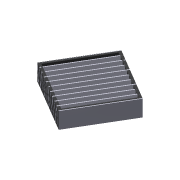
# Autodesk Inventor part: filter ver1
Saved by Autodesk Inventor 2016 (Build 200138000, 138)
## iProperties
Created: 2018-02-22
Part Number: filter ver1
Material: Generic
Document SubType Name: Modeling
Designer: Juny
Density: 1 g/cm^3
Appearance: Default
Author: Juny
Autodesk Inventor part; units mm, degrees
ref_plane "YZ Plane" through (0, 0, 0) normal (1, 0, 0) x (0, 1, 0)
ref_plane "XZ Plane" through (0, 0, 0) normal (0, 1, 0) x (-1, 0, 0)
ref_plane "XY Plane" through (0, 0, 0) normal (0, 0, 1) x (1, 0, 0)
sketch "Sketch1" plane through (0, 0, 0) normal (0, 0, 1) x (1, 0, 0)
  line L0 (22.5214, 7.9449) -> (30.3551, 21.1573) projected
  ellipse E0 centre (32.9355, 19.6263) end of major axis (32.1925, 22.5337) minor radius 3 (34.465, 22.2076) -> (30.3551, 21.1573) ccw projected
  line L1 (34.465, 22.2076) -> (47.6774, 14.3739) projected
  ellipse E1 centre (46.1463, 11.7935) end of major axis (49.0538, 12.5365) minor radius 3 (48.7277, 10.264) -> (47.6774, 14.3739) ccw projected
  line L2 (48.7277, 10.264) -> (40.894, -2.9483) projected
  ellipse E2 centre (38.3136, -1.4173) end of major axis (39.0566, -4.3248) minor radius 3 (36.7841, -3.9987) -> (40.894, -2.9483) ccw projected
  line L3 (36.7841, -3.9987) -> (23.5717, 3.835) projected
  ellipse E3 centre (25.1028, 6.4154) end of major axis (22.1953, 5.6724) minor radius 3 (22.5214, 7.9449) -> (23.5717, 3.835) ccw projected
  line L4 (9.2613, -14.4196) -> (17.095, -1.2072) projected
  ellipse E4 centre (19.6755, -2.7383) end of major axis (18.9324, 0.1692) minor radius 3 (21.2049, -0.1569) -> (17.095, -1.2072) ccw projected
  line L5 (21.2049, -0.1569) -> (34.4173, -7.9906) projected
  ellipse E5 centre (32.8863, -10.571) end of major axis (35.7938, -9.828) minor radius 3 (35.4677, -12.1005) -> (34.4173, -7.9906) ccw projected
  line L6 (35.4677, -12.1005) -> (27.634, -25.3129) projected
  ellipse E6 centre (25.0535, -23.7818) end of major axis (25.7966, -26.6893) minor radius 3 (23.5241, -26.3632) -> (27.634, -25.3129) ccw projected
  line L7 (23.5241, -26.3632) -> (10.3117, -18.5295) projected
  ellipse E7 centre (11.8427, -15.9491) end of major axis (8.9353, -16.6921) minor radius 3 (9.2613, -14.4196) -> (10.3117, -18.5295) ccw projected
  line L8 (-3.9987, -36.7841) -> (3.835, -23.5717) projected
  ellipse E8 centre (6.4154, -25.1028) end of major axis (5.6724, -22.1953) minor radius 3 (7.9449, -22.5214) -> (3.835, -23.5717) ccw projected
  line L9 (7.9449, -22.5214) -> (21.1573, -30.3551) projected
  ellipse E9 centre (19.6263, -32.9355) end of major axis (22.5337, -32.1925) minor radius 3 (22.2076, -34.465) -> (21.1573, -30.3551) ccw projected
  line L10 (22.2076, -34.465) -> (14.3739, -47.6774) projected
  ellipse E10 centre (11.7935, -46.1463) end of major axis (12.5365, -49.0538) minor radius 3 (10.264, -48.7277) -> (14.3739, -47.6774) ccw projected
  line L11 (10.264, -48.7277) -> (-2.9483, -40.894) projected
  ellipse E11 centre (-1.4173, -38.3136) end of major axis (-4.3248, -39.0566) minor radius 3 (-3.9987, -36.7841) -> (-2.9483, -40.894) ccw projected
  line L12 (0.1569, 21.2049) -> (7.9906, 34.4173) projected
  ellipse E12 centre (10.571, 32.8863) end of major axis (9.828, 35.7938) minor radius 3 (12.1005, 35.4677) -> (7.9906, 34.4173) ccw projected
  line L13 (12.1005, 35.4677) -> (25.3129, 27.634) projected
  ellipse E13 centre (23.7818, 25.0535) end of major axis (26.6893, 25.7966) minor radius 3 (26.3632, 23.5241) -> (25.3129, 27.634) ccw projected
  line L14 (26.3632, 23.5241) -> (18.5295, 10.3117) projected
  ellipse E14 centre (15.9491, 11.8427) end of major axis (16.6921, 8.9353) minor radius 3 (14.4196, 9.2613) -> (18.5295, 10.3117) ccw projected
  line L15 (14.4196, 9.2613) -> (1.2072, 17.095) projected
  ellipse E15 centre (2.7383, 19.6755) end of major axis (-0.1692, 18.9324) minor radius 3 (0.1569, 21.2049) -> (1.2072, 17.095) ccw projected
  line L16 (-13.1032, -1.1596) -> (-5.2695, 12.0528) projected
  ellipse E16 centre (-2.689, 10.5218) end of major axis (-3.4321, 13.4293) minor radius 3 (-1.1596, 13.1032) -> (-5.2695, 12.0528) ccw projected
  line L17 (-1.1596, 13.1032) -> (12.0528, 5.2695) projected
  ellipse E17 centre (10.5218, 2.689) end of major axis (13.4293, 3.4321) minor radius 3 (13.1032, 1.1596) -> (12.0528, 5.2695) ccw projected
  line L18 (13.1032, 1.1596) -> (5.2695, -12.0528) projected
  ellipse E18 centre (2.689, -10.5218) end of major axis (3.4321, -13.4293) minor radius 3 (1.1596, -13.1032) -> (5.2695, -12.0528) ccw projected
  line L19 (1.1596, -13.1032) -> (-12.0528, -5.2695) projected
  ellipse E19 centre (-10.5218, -2.689) end of major axis (-13.4293, -3.4321) minor radius 3 (-13.1032, -1.1596) -> (-12.0528, -5.2695) ccw projected
  line L20 (-26.3632, -23.5241) -> (-18.5295, -10.3117) projected
  ellipse E20 centre (-15.9491, -11.8427) end of major axis (-16.6921, -8.9353) minor radius 3 (-14.4196, -9.2613) -> (-18.5295, -10.3117) ccw projected
  line L21 (-14.4196, -9.2613) -> (-1.2072, -17.095) projected
  ellipse E21 centre (-2.7383, -19.6755) end of major axis (0.1692, -18.9324) minor radius 3 (-0.1569, -21.2049) -> (-1.2072, -17.095) ccw projected
  line L22 (-0.1569, -21.2049) -> (-7.9906, -34.4173) projected
  ellipse E22 centre (-10.571, -32.8863) end of major axis (-9.828, -35.7938) minor radius 3 (-12.1005, -35.4677) -> (-7.9906, -34.4173) ccw projected
  line L23 (-12.1005, -35.4677) -> (-25.3129, -27.634) projected
  ellipse E23 centre (-23.7818, -25.0535) end of major axis (-26.6893, -25.7966) minor radius 3 (-26.3632, -23.5241) -> (-25.3129, -27.634) ccw projected
  line L24 (-22.2076, 34.465) -> (-14.3739, 47.6774) projected
  ellipse E24 centre (-11.7935, 46.1463) end of major axis (-12.5365, 49.0538) minor radius 3 (-10.264, 48.7277) -> (-14.3739, 47.6774) ccw projected
  line L25 (-10.264, 48.7277) -> (2.9483, 40.894) projected
  ellipse E25 centre (1.4173, 38.3136) end of major axis (4.3248, 39.0566) minor radius 3 (3.9987, 36.7841) -> (2.9483, 40.894) ccw projected
  line L26 (3.9987, 36.7841) -> (-3.835, 23.5717) projected
  ellipse E26 centre (-6.4154, 25.1028) end of major axis (-5.6724, 22.1953) minor radius 3 (-7.9449, 22.5214) -> (-3.835, 23.5717) ccw projected
  line L27 (-7.9449, 22.5214) -> (-21.1573, 30.3551) projected
  ellipse E27 centre (-19.6263, 32.9355) end of major axis (-22.5337, 32.1925) minor radius 3 (-22.2076, 34.465) -> (-21.1573, 30.3551) ccw projected
  line L28 (-35.4677, 12.1005) -> (-27.634, 25.3129) projected
  ellipse E28 centre (-25.0535, 23.7818) end of major axis (-25.7966, 26.6893) minor radius 3 (-23.5241, 26.3632) -> (-27.634, 25.3129) ccw projected
  line L29 (-23.5241, 26.3632) -> (-10.3117, 18.5295) projected
  ellipse E29 centre (-11.8427, 15.9491) end of major axis (-8.9353, 16.6921) minor radius 3 (-9.2613, 14.4196) -> (-10.3117, 18.5295) ccw projected
  line L30 (-9.2613, 14.4196) -> (-17.095, 1.2072) projected
  ellipse E30 centre (-19.6755, 2.7383) end of major axis (-18.9324, -0.1692) minor radius 3 (-21.2049, 0.1569) -> (-17.095, 1.2072) ccw projected
  line L31 (-21.2049, 0.1569) -> (-34.4173, 7.9906) projected
  ellipse E31 centre (-32.8863, 10.571) end of major axis (-35.7938, 9.828) minor radius 3 (-35.4677, 12.1005) -> (-34.4173, 7.9906) ccw projected
  line L32 (-48.7277, -10.264) -> (-40.894, 2.9483) projected
  ellipse E32 centre (-38.3136, 1.4173) end of major axis (-39.0566, 4.3248) minor radius 3 (-36.7841, 3.9987) -> (-40.894, 2.9483) ccw projected
  line L33 (-36.7841, 3.9987) -> (-23.5717, -3.835) projected
  ellipse E33 centre (-25.1028, -6.4154) end of major axis (-22.1953, -5.6724) minor radius 3 (-22.5214, -7.9449) -> (-23.5717, -3.835) ccw projected
  line L34 (-22.5214, -7.9449) -> (-30.3551, -21.1573) projected
  ellipse E34 centre (-32.9355, -19.6263) end of major axis (-32.1925, -22.5337) minor radius 3 (-34.465, -22.2076) -> (-30.3551, -21.1573) ccw projected
  line L35 (-34.465, -22.2076) -> (-47.6774, -14.3739) projected
  ellipse E35 centre (-46.1463, -11.7935) end of major axis (-49.0538, -12.5365) minor radius 3 (-48.7277, -10.264) -> (-47.6774, -14.3739) ccw projected
  line L36 (-51.6751, -13.2065) -> (-13.2065, 51.6751) projected
  line L37 (13.2065, -51.6751) -> (-51.6751, -13.2065) projected
  line L38 (51.6751, 13.2065) -> (13.2065, -51.6751) projected
  line L39 (-13.2065, 51.6751) -> (51.6751, 13.2065) projected
  point P0 (0, 0)
  constraints: 36 other
extrude "Extrusion1" add sketch "Sketch1" along normal blind 20 contours L0 E0 L1 E1 L2 E2 L3 E3 | L4 E4 L5 E5 L6 E6 L7 E7 | L8 E8 L9 E9 L10 E10 L11 E11 | L12 E12 L13 E13 L14 E14 L15 E15 | L16 E16 L17 E17 L18 E18 L19 E19 | L20 E20 L21 E21 L22 E22 L23 E23 | L24 E24 L25 E25 L26 E26 L27 E27 | L28 E28 L29 E29 L30 E30 L31 E31 | L32 E32 L33 E33 L34 E34 L35 E35 | L36 L39 L38 L37
sketch "Sketch2" plane through (-13.2065, 51.6751, 20) normal (0.5100017, 0.8601734, 0) x (0.8601734, -0.5100017, 0)
  line L0 (0, 20) -> (75.4284, 20) projected
  line L1 (0, 20) -> (0, 0) projected
  line L2 (75.4284, 0) -> (0, 0) projected
  line L3 (75.4284, 20) -> (75.4284, 0) projected
  line L4 (75.4284, 0) -> (0, 0) projected
  line L5 (74.4284, 0) -> (71.2545, 18)
  line L6 (71.2545, 18) -> (68.0807, 0)
  line L7 (70.5918, 20) -> (67.4179, 2)
  line L8 (67.4179, 2) -> (64.244, 20)
  line L9 (0, 20) -> (75.4284, 20) projected
  point P0 (37.7142, 20)
  dimension "d2" = 20
  dimension "d3" = 10
  dimension "d4" = 2
  dimension "d5" = 20
  dimension "d6" = 1
  dimension "d7" = 2
  dimension "d8" = 1
  constraints: 8 end point, 4 point on line, 1 parallel
  measures "d2" angle of L6 L5
  measures "d3" angle of L3 L5
  measures "d4" distance from line of L0 L5.end
  measures "d5" angle of L8 L7
  measures "d6" distance between parallel lines of L6 L7
  measures "d7" distance from line of L2 L7.end
  measures "d8" distance from line of L3 L5.start
extrude "Extrusion2" cut sketch "Sketch2" against normal blind 100 contours L0 L7 L8 | L6 L5 L2
pattern_linear "Rectangular Pattern1" count 10 spacing 7.5 along (-0.8601734, 0.5100017, 0) of "Extrusion2"
sketch "Sketch3" plane through (0, 0, 20) normal (0, 0, 1) x (1, 0, 0)
  line L0 (50.8149, 13.7165) -> (12.3463, -51.1651) projected
  line L1 (12.3463, -51.1651) -> (13.2065, -51.6751) projected
  line L2 (13.2065, -51.6751) -> (51.6751, 13.2065) projected
  line L3 (51.6751, 13.2065) -> (50.8149, 13.7165) projected
  line L4 (-51.1756, -13.5026) -> (-12.707, 51.3789) projected
  line L5 (-12.707, 51.3789) -> (-13.2065, 51.6751) projected
  line L6 (-13.2065, 51.6751) -> (-51.6751, -13.2065) projected
  line L7 (-51.6751, -13.2065) -> (-51.1756, -13.5026) projected
  line L8 (-13.2065, 51.6751) -> (-51.6751, -13.2065) projected
  line L9 (-13.2065, 51.6751) -> (-51.6751, -13.2065)
  line L10 (-51.6751, -13.2065) -> (13.2065, -51.6751)
  line L11 (13.2065, -51.6751) -> (51.6751, 13.2065)
  line L12 (51.6751, 13.2065) -> (-13.2065, 51.6751)
  line L13 (12.1559, -47.5646) -> (-47.5646, -12.1559)
  line L14 (-47.5646, -12.1559) -> (-12.1559, 47.5646)
  line L15 (-12.1559, 47.5646) -> (47.5646, 12.1559)
  line L16 (47.5646, 12.1559) -> (12.1559, -47.5646)
  point P0 (0, 0)
  dimension "d14" = 3
  constraints: 16 end point, 5 equal length, 2 perpendicular, 3 other
  measures "d14" distance between parallel lines of L10 L13
extrude "Extrusion3" add sketch "Sketch3" against normal blind 20 separate body
body "Solid1"
body "Solid2"
